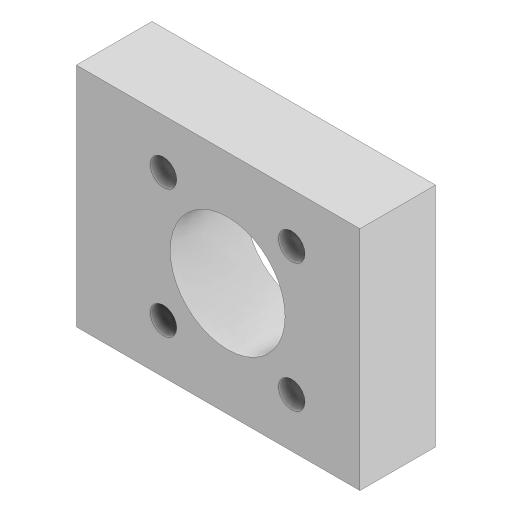
# Autodesk Inventor part: POSIBLE CORTE
Saved by Autodesk Inventor 2024 (Build 280153000, 153)
## iProperties
Created: 2024-06-27
Part Number: POSIBLE CORTE
Material: Generic
Document SubType Name: Modeling
Designer: Jhuliams
Density: 1 g/cm^3
Appearance: Default
Author: Jhuliams
Autodesk Inventor part; units mm, degrees
ref_plane "YZ Plane" through (0, 0, 0) normal (1, 0, 0) x (0, 1, 0)
ref_plane "XZ Plane" through (0, 0, 0) normal (0, 1, 0) x (-1, 0, 0)
ref_plane "XY Plane" through (0, 0, 0) normal (0, 0, 1) x (1, 0, 0)
sketch "Sketch1" plane through (0, 0, 0) normal (0, 0, 1) x (1, 0, 0)
  line L0 (-18.75, 15) -> (18.75, 15)
  line L1 (18.75, 15) -> (18.75, -15)
  line L2 (18.75, -15) -> (-18.75, -15)
  line L3 (-18.75, -15) -> (-18.75, 15)
  line L4 (-18.75, 15) -> (18.75, -15) construction
  line L5 (18.75, 15) -> (-18.75, -15) construction
  line L6 (18.75, 0) -> (1.25, 0)
  circle A0 centre (1.25, 0) radius 7.6
  circle A1 centre (1.25, 0) radius 12
  line L7 (-11.25, 12.5) -> (13.75, 12.5)
  line L8 (13.75, 12.5) -> (13.75, -12.5)
  line L9 (13.75, -12.5) -> (-11.25, -12.5)
  line L10 (-11.25, -12.5) -> (-11.25, 12.5)
  line L11 (-11.25, 12.5) -> (13.75, -12.5) construction
  line L12 (13.75, 12.5) -> (-11.25, -12.5) construction
  line L13 (13.75, 12.5) -> (-11.25, -12.5)
  circle A2 centre (9.7353, 8.4853) radius 1.75
  circle A3 centre (-7.2353, 8.4853) radius 1.75
  circle A4 centre (-7.2353, -8.4853) radius 1.75
  circle A5 centre (9.7353, -8.4853) radius 1.75
  point P0 (0, 0)
  dimension "d4" = 24
  dimension "d0" = 37.5
  dimension "d1" = 30
  dimension "d2" = 17.5
  dimension "d3" = 15.2
  dimension "d5" = 25
  dimension "d6" = 25
  dimension "d7" = 3.5
  dimension "d10" = 360
  constraints: 28 end point, 5 centre point, 5 midpoint, 4 parallel, 3 horizontal, 2 coincident, 2 perpendicular, 1 point on line, 12 other
  measures "d0" distance of L1.end L2.end
  measures "d1" distance of L0.end L1.end
  measures "d2" distance of L6.start L6.end
  measures "d3" diameter of A0
  measures "d5" distance of L8.end L9.end
  measures "d6" distance of L7.end L8.end
  measures "d7" diameter of A2
extrude "Extrusion1" add sketch "Sketch1" along normal blind 10 contours L8 L9 L13 A4 A1 A5 L6 | L6 A1 A2 L13 L8 | L0 L1 L2 L3 | A1 A5 A4 L13 A0 L6 | L6 A0 L13 A2 A1 | L13 A2 A1 A3 A4 L10 L7 | A0 L13 A4 A1 A3 A2
body "Solid1"
